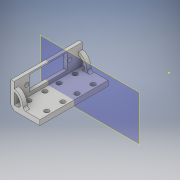
# Autodesk Inventor part: x_carriage_to_extruder
Saved by Autodesk Inventor 2019 (Build 230136000, 136)
## iProperties
Created: 2020-04-12
Part Number: x_carriage_to_extruder
Material: Generisch
Document SubType Name: Modeling
Designer: marc
Density: 1 g/cm^3
Appearance: Vorgabe
Author: marc
## iProperties of the stored document plug_3D-Druck.ipt
Created: 2020-04-26
Part Number: plug_3D-Druck
Material: Generisch
Document SubType Name: Modeling
Designer: marc
Density: 1 g/cm^3
Appearance: Vorgabe
Author: marc
Autodesk Inventor part; units mm, degrees
ref_plane "YZ Plane" through (0, 0, 0) normal (1, 0, 0) x (0, 1, 0)
ref_plane "XZ Plane" through (0, 0, 0) normal (0, 1, 0) x (-1, 0, 0)
ref_plane "XY Plane" through (0, 0, 0) normal (0, 0, 1) x (1, 0, 0)
sketch "Skizze1" plane through (0, 0, 0) normal (0, 1, 0) x (-1, 0, 0)
  line L0 (0, 0) -> (70, 0)
  line L1 (70, 0) -> (70, 53)
  line L2 (0, 6) -> (0, 0)
  line L3 (70, 53) -> (0, 53)
  line L4 (0, 53) -> (0, 47)
  line L5 (0, 47) -> (64, 47)
  line L6 (64, 47) -> (64, 6)
  line L7 (64, 6) -> (0, 6)
  dimension "d4" = 53
  dimension "d5" = 6
  dimension "d6" = 6
  dimension "d7" = 70
  dimension "d8" = 6
  constraints: 16 end point, 4 perpendicular, 2 horizontal, 1 parallel, 1 vertical, 1 vertical alignment
  measures "d4" distance between parallel lines of L0 L3
  measures "d5" distance of L2.start L0.start
  measures "d6" distance between parallel lines of L1 L6
  measures "d7" distance of L0.start L0.end
  measures "d8" distance of L3.end L4.end
extrude "Extrusion1" add sketch "Skizze1" along normal blind 4
sketch "Skizze2" plane through (0, 4, 0) normal (0, 1, 0) x (1, 0, 0)
  point P0 (0, 0)
sketch "Skizze3" plane through (-70, 0, 53) normal (0, 0, 1) x (1, 0, 0)
  line L0 (70, 0) -> (0, 0) projected
  line L1 (25, 0) -> (50, 0)
  line L2 (50, 0) -> (50, 1.8)
  line L3 (50, 1.8) -> (25, 1.8)
  line L4 (25, 1.8) -> (25, 0)
  line L5 (70, 0) -> (70, 4) projected
  dimension "d11" = 1.8
  dimension "d12" = 25
  dimension "d13" = 20
  constraints: 8 end point, 2 parallel, 1 horizontal, 1 perpendicular, 1 point on line
  measures "d11" distance of L1.end L2.end
  measures "d12" distance of L2.end L3.end
  measures "d13" distance between parallel lines of L5 L2
extrude "Extrusion2" cut sketch "Skizze3" against normal up to surface (6 mm away)
sketch "Skizze4" plane through (0, 4, 0) normal (0, 1, 0) x (1, 0, 0)
  line L0 (0, -53) -> (0, -47) projected
  line L1 (-70, -53) -> (0, -53) projected
  line L2 (-64, -6) -> (0, -6) projected
  point P0 (0, 0)
  point P1 (-3, -50)
  point P2 (-3, -3)
  point P3 (-60, -50)
  point P4 (-60, -3)
  point P5 (-50, -3)
  point P6 (-50, -50)
  point P7 (-13, -50)
  point P8 (-13, -3)
  dimension "d20" = 3
  dimension "d21" = 3
  dimension "d22" = 6
  dimension "d23" = 3
  dimension "d24" = 10
  dimension "d25" = 37
  dimension "d26" = 10
  constraints: 6 horizontal alignment, 4 vertical alignment
  measures "d20" distance from line of L0 point (-3, -50)
  measures "d21" distance from line of L1 point (-3, -50)
  measures "d22" distance of L0.start L0.end
  measures "d23" distance from line of L2 point (-3, -3)
  measures "d24" distance of point (-3, -50) point (-13, -50)
  measures "d25" distance of point (-50, -50) point (-13, -50)
  measures "d26" distance of point (-50, -50) point (-60, -50)
hole "Bohrung1" at (-60, 4, 50) at (-50, 4, 50) at (-13, 4, 50) at (-3, 4, 50) at (-3, 4, 3) at (-13, 4, 3) at (-50, 4, 3) at (-60, 4, 3) direction (0, -1, 0) diameter 3.6 end through all clearance for "Flachkopfsenkschraube DIN EN ISO 2009" size "M3" standard "DIN"
chamfer "Fase2" distance 1 angle 45 2 edges at (0, 4, 50) (0, 4, 3)
sketch "Skizze6" plane through (0, 0, 0) normal (0, -1, 0) x (1, 0, 0)
  line L0 (-64, 6) -> (-1, 6) projected
  line L1 (-64, 6) -> (-64, 0)
  line L2 (-1, 0) -> (-70, 0) projected
  line L3 (-1, 47) -> (-64, 47) projected
  line L4 (-64, 47) -> (-64, 53)
  line L5 (-70, 53) -> (-1, 53) projected
  line L6 (-64, 47) -> (-64, 6) projected
  line L7 (-70, 0) -> (-70, 53) projected
  point P0 (0, 0)
  constraints: 4 end point, 3 point on line, 1 vertical
extrude "Extrusion3" add sketch "Skizze6" along normal blind 25
sketch "Skizze8" plane through (0, -25, 0) normal (0, -1, 0) x (1, 0, 0)
  line L0 (-70, 0) -> (-70, 53) projected
  line L1 (-70, 53) -> (-54, 53)
  line L2 (-54, 53) -> (-54, 0)
  line L3 (-54, 0) -> (-70, 0)
  line L4 (-70, 0) -> (-70, 53)
  point P0 (0, 0)
  dimension "d40" = 16
  constraints: 8 end point, 2 parallel, 1 horizontal, 1 perpendicular, 1 point on line
  measures "d40" distance of L2.end L3.end
extrude "Extrusion4" add sketch "Skizze8" along normal blind 3
move faces "Verschieben1" translate (6.5, 0, 0) faces at (-54, -27, 17.6667)
sketch "Skizze9" plane through (0, -28, 0) normal (0, -1, 0) x (1, 0, 0)
  line L0 (-70, 53) -> (-70, 0) projected
  line L1 (-47.5, 53) -> (-70, 53) projected
  point P0 (0, 0)
  point P1 (-64.6, 8.5)
  point P2 (-64.6, 21)
  point P3 (-64.6, 32)
  point P4 (-64.6, 44.5)
  point P5 (-50.6, 21)
  point P6 (-50.6, 8.5)
  point P7 (-50.6, 32)
  point P8 (-50.6, 44.5)
  dimension "d43" = 5.4
  dimension "d44" = 12.5
  dimension "d45" = 14
  dimension "d49" = 12.5
  dimension "d50" = 11
  dimension "d51" = 53
  dimension "d52" = 36
  dimension "d53" = 8.5
  constraints: 6 vertical alignment, 4 horizontal alignment
  measures "d43" distance from line of L0 point (-64.6, 21)
  measures "d44" distance of point (-64.6, 8.5) point (-64.6, 21)
  measures "d45" distance of point (-50.6, 21) point (-64.6, 21)
  measures "d49" distance of point (-64.6, 44.5) point (-64.6, 32)
  measures "d50" distance of point (-64.6, 21) point (-64.6, 32)
  measures "d51" distance of L0.start L0.end
  measures "d52" distance of point (-64.6, 8.5) point (-64.6, 44.5)
  measures "d53" distance from line of L1 point (-64.6, 44.5)
hole "Bohrung2" at (-50.6, -28, 8.5) at (-50.6, -28, 21) at (-64.6, -28, 8.5) at (-64.6, -28, 21) at (-50.6, -28, 32) at (-50.6, -28, 44.5) at (-64.6, -28, 44.5) at (-64.6, -28, 32) direction (0, 1, 0) diameter 3.6 end through all clearance for "Flachkopfsenkschraube DIN EN ISO 2009" size "M3" standard "DIN"
sketch "Skizze12" plane through (0, 4, 0) normal (0, 1, 0) x (1, 0, 0)
  line L0 (-61.75, -6.8546) -> (-61.75, -10.1454) projected
  line L1 (-67.45, -42.8546) -> (-64.6, -41.2091) projected
  line L2 (-61.75, -10.1454) -> (-67.45, -10.1454)
  line L3 (-67.45, -10.1454) -> (-67.45, -42.8546)
  line L4 (-67.45, -42.8546) -> (-61.75, -42.8546)
  line L5 (-61.75, -42.8546) -> (-61.75, -10.1454)
  point P0 (0, 0)
  constraints: 8 end point, 2 parallel, 1 horizontal, 1 perpendicular
extrude "Extrusion6" cut sketch "Skizze12" against normal up to surface (29 mm away)
chamfer "Fase3" distance 1.7 angle 45 2 edges at (-20, 1.8, 50) (-45, 1.8, 50)
fillet "Rundung1" radius 2 2 edges at (-20, 0, 50) (-45, 0, 50)
chamfer "Fase4" distance 1.7 angle 45 2 edges at (-70, -28, 26.5) (-70, 4, 26.5)
sketch "Skizze17" plane through (0, 0, 53) normal (0, 0, 1) x (1, 0, 0)
  line L0 (-46.2285, 0) -> (0, 0)
  line L1 (0, 0) -> (0, 4)
  line L2 (0, 4) -> (-46.2285, 4)
  line L3 (-46.2285, 4) -> (-46.2285, 0)
  line L4 (-64, 0) -> (-45.6245, 0) projected
  point P0 (0, 0)
  point P1 (-1, 4)
  dimension "d98" = 46.2285
  constraints: 8 end point, 4 point on line, 2 parallel, 1 horizontal, 1 perpendicular
  measures "d98" distance of L1.end L2.end
extrude "Extrusion9" cut sketch "Skizze17" against normal up to surface (6 mm away)
sketch "Skizze21" plane through (0, 4, 0) normal (0, 1, 0) x (1, 0, 0)
  point P0 (0, 0)
sketch "Skizze22" plane through (0, 4, 0) normal (0, 1, 0) x (1, 0, 0)
  line L0 (-72.329, -54.114) -> (1.2728, -54.114)
  line L1 (1.2728, -54.114) -> (1.2728, 2.5028)
  line L2 (1.2728, 2.5028) -> (-72.329, 2.5028)
  line L3 (-72.329, 2.5028) -> (-72.329, -54.114)
  point P0 (0, 0)
  constraints: 8 end point, 2 parallel, 1 horizontal, 1 perpendicular
extrude "Extrusion12" cut sketch "Skizze22" against normal blind 13.25
sketch "Skizze24" plane through (-67.45, -25, 10.1454) normal (0, 0, 1) x (1, 0, 0)
  line L0 (0, 0) -> (14.6962, 0)
  line L1 (14.6962, 0) -> (14.6962, 12.391)
  line L2 (14.6962, 12.391) -> (0, 12.391)
  line L3 (0, 12.391) -> (0, 0)
  point P0 (67.45, 25)
  constraints: 8 end point, 2 parallel, 1 horizontal, 1 perpendicular
extrude "Extrusion13" cut sketch "Skizze24" against normal blind 18.25
sketch "Skizze25" plane through (-65.3297, -25, 42.8546) normal (0, 0, -1) x (-1, 0, 0)
  line L0 (2.1203, 15.75) -> (2.1203, 0) projected
  line L1 (2.1203, 0) -> (-4.7793, 0)
  line L2 (-4.7793, 0) -> (-4.7793, 14.0736)
  line L3 (-4.7793, 14.0736) -> (2.1203, 14.0736)
  line L4 (2.1203, 14.0736) -> (2.1203, 0)
  point P0 (-65.3297, 25)
  constraints: 8 end point, 2 parallel, 1 horizontal, 1 perpendicular
extrude "Extrusion14" cut sketch "Skizze25" against normal blind 18.25
sketch "Skizze26" plane through (-67.45, -25, 53) normal (1, 0, 0) x (0, 0, -1)
  circle A0 centre (43.25, 8.7132) radius 1.6
  circle A1 centre (9.75, 8.7132) radius 1.6
  line L0 (0, 0) -> (0, 14.0736) projected
  line L1 (53, 12.391) -> (53, 0) projected
  line L2 (42.8546, 15.75) -> (10.1454, 15.75) projected
  line L3 (41.15, 2.7132) -> (11.85, 2.7132)
  line L4 (11.85, 2.7132) -> (11.85, 14.7132)
  line L5 (11.85, 14.7132) -> (41.15, 14.7132)
  line L6 (41.15, 14.7132) -> (41.15, 2.7132)
  point P0 (53, 25)
  point P1 (0, 10.75)
  point P2 (53, 10.75)
  point P3 (10.1454, 15.75)
  dimension "d135" = 3.2
  dimension "d136" = 3.2
  dimension "d137" = 33.5
  dimension "d138" = 9.75
  dimension "d139" = 53
  dimension "d140" = 7.0368
  dimension "d142" = 2.1
  dimension "d143" = 2.1
  dimension "d144" = 12
  dimension "d145" = 1.0368
  dimension "d162" = 14.0736
  constraints: 8 end point, 2 centre point, 2 parallel, 1 horizontal, 1 horizontal alignment, 1 perpendicular, 1 other
  measures "d135" diameter of A0
  measures "d136" diameter of A1
  measures "d137" distance of A0.centre A1.centre
  measures "d138" distance from line of L0 A1.centre
  measures "d139" distance between parallel lines of L0 L1
  measures "d142" distance from line of L6 A0.centre
  measures "d143" distance from line of L4 A1.centre
  measures "d144" distance between parallel lines of L5 L3
  measures "d162" distance of L0.start L0.end
extrude "Extrusion15" cut sketch "Skizze26" against normal blind 18.25
sketch "Skizze27" plane through (-47.5, -28, 0) normal (0, 0, -1) x (-1, 0, 0)
  line L0 (19.95, 15.391) -> (19.95, 3) projected
  ellipse E0 centre (19.95, 3) end of major axis (19.95, 13.75) minor radius 7 (19.95, 13.75) -> (12.95, 3) ccw
  ellipse E1 centre (19.95, 3) end of major axis (19.95, 11.5) minor radius 5 (19.95, 11.5) -> (14.95, 3) ccw
  line L1 (14.95, 3) -> (12.95, 3)
  line L2 (0, 3) -> (19.95, 3) projected
  line L3 (19.95, 11.5) -> (19.95, 13.75)
  point P0 (-47.5, 28)
  dimension "d148" = 7
  dimension "d149" = 5
  dimension "d151" = 2
  dimension "d161" = 2.25
  constraints: 4 end point, 2 coincident, 2 point on line, 1 collinear, 1 horizontal alignment, 8 other
  measures "d151" distance of L1.start L1.end
  measures "d161" distance of L3.start L3.end
extrude "Extrusion16" add sketch "Skizze27" against normal blind 3.25 contours L0 E1 L1 E0
ref_plane "Arbeitsebene2" through (-47.5, -28, 26.5) normal (0, 0, -1) x (-1, 0, 0)
mirror "Spiegeln2" about plane through (-47.5, -28, 26.5) normal (0, 0, -1) of "Extrusion16"
move faces "Verschieben2" translate (0, -1, 0) faces at (-59.8545, -28, 2.3021)
fillet "Rundung3" radius 2 4 edges at (-60.45, -25, 1.625) (-60.45, -25, 51.375) (-62.45, -25, 51.375) (-62.45, -25, 1.625)
sketch "Skizze28" plane through (-67.45, -12.609, 10.1454) normal (0, -1, 0) x (1, 0, 0)
  line L0 (0, -10.1454) -> (33.6242, -10.1454)
  line L1 (33.6242, -10.1454) -> (33.6242, 52.2462)
  line L2 (33.6242, 52.2462) -> (0, 52.2462)
  line L3 (0, 52.2462) -> (0, -10.1454)
  line L4 (3.45, -10.1454) -> (0, -10.1454) projected
  point P0 (67.45, -10.1454)
  constraints: 8 end point, 4 coincident, 2 parallel, 1 horizontal, 1 perpendicular
extrude "Extrusion17" cut sketch "Skizze28" against normal blind 11.25
equation "\"d6\" = d5"
equation "\"d21\" = 0.5 * d22"
equation "\"d23\" = d21"
equation "\"d49\" = d44"
equation "\"d53\" = -0.5 * d52 + 0.5 * d51"
equation "\"d136\" = d135"
equation "\"d138\" = -0.5 * d137 + 0.5 * d139"
equation "\"d140\" = 0.5 * d162"
equation "\"d143\" = d142"
equation "\"d145\" = -0.5 * d144 + 0.5 * d162"
